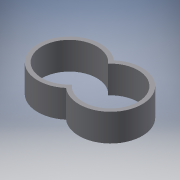
# Autodesk Inventor part: housing
Saved by Autodesk Inventor 2018.3 (Build 223284000, 284)
## iProperties
Created: 2021-03-20
Part Number: housing
Material: Generic
Document SubType Name: Modeling
Designer: kenbl
Density: 1 g/cm^3
Appearance: Default
Author: kenbl
Autodesk Inventor part; units mm, degrees
ref_plane "YZ Plane" through (0, 0, 0) normal (1, 0, 0) x (0, 1, 0)
ref_plane "XZ Plane" through (0, 0, 0) normal (0, 1, 0) x (-1, 0, 0)
ref_plane "XY Plane" through (0, 0, 0) normal (0, 0, 1) x (1, 0, 0)
sketch "Sketch1" plane through (0, 0, 0) normal (0, 0, 1) x (1, 0, 0)
  arc A0 (0, 13.143225) -> (0, -13.143225) centre (-15.075, 0) ccw
  arc A1 (0, -13.143225) -> (0, 13.143225) centre (15.075, 0) ccw
  line L0 (-15.075, 0) -> (15.075, 0)
  arc A2 (0, -17.370791) -> (0, 17.370791) centre (-15.075, 0) ccw construction
  arc A3 (0, 17.370791) -> (0, -17.370791) centre (15.075, 0) ccw construction
  arc A4 (0, -17.370791) -> (0, 17.370791) centre (15.075, 0) ccw
  arc A5 (0, 17.370791) -> (0, -17.370791) centre (-15.075, 0) ccw
  arc A6 (0, 13.143225) -> (0, -13.143225) centre (15.075, 0) ccw construction
  arc A7 (0, -13.143225) -> (0, 13.143225) centre (-15.075, 0) ccw construction
  point P0 (0, 0)
  point P1 (0, 0)
  dimension "d0" = 40
  dimension "d1" = 30.15
  dimension "d2" = 3
  dimension "d3" = 3
  constraints: 16 point on circle, 8 centre point, 3 coincident, 2 end point, 1 equal radius, 1 horizontal, 1 midpoint
  measures "d0" diameter of A0
  measures "d1" distance of L0.start L0.end
  measures "d2" radial gap between concentric circles of A0 A2
  measures "d3" radial gap between concentric circles of A3 A1
extrude "Extrusion1" add sketch "Sketch1" along normal blind 20
thicken "Thicken1" operation add thickness 0.15 both sides no extend neighbours yes toward (0.0352431, -0.9993788, 0) faces at (15.779861, -19.987575, 6.666667) (-15.779861, 19.987575, 6.666667)
equation "\"d3\" = d2"
equation "\"d6\" = tol"
equation "\"d7\" = 0.5 * tol"
equation "\"tol\" = 0.15"
body "Solid1"
